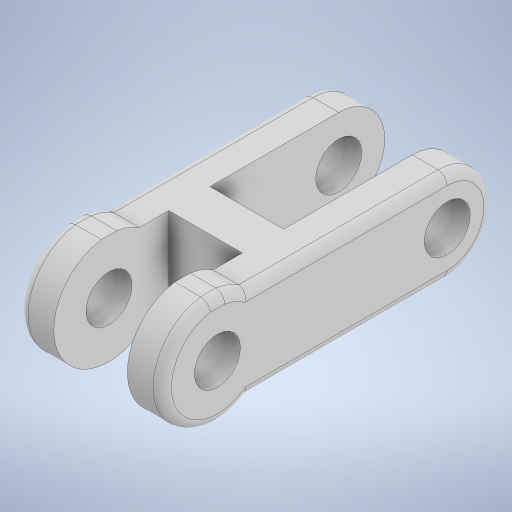
# Autodesk Inventor part: part2
Saved by Autodesk Inventor 2024 (Build 280153000, 153)
## iProperties
Created: 2023-08-22
Part Number: part2
Material: Generic
Document SubType Name: Modeling
Designer: admins
Density: 1 g/cm^3
Appearance: Default
Author: admins
Autodesk Inventor part; units mm, degrees
ref_plane "YZ Plane" through (0, 0, 0) normal (1, 0, 0) x (0, 1, 0)
ref_plane "XZ Plane" through (0, 0, 0) normal (0, 1, 0) x (-1, 0, 0)
ref_plane "XY Plane" through (0, 0, 0) normal (0, 0, 1) x (1, 0, 0)
sketch "Sketch1" plane through (0, 0, 0) normal (0, 1, 0) x (-1, 0, 0)
  line L0 (-138.4477, 131.5515) -> (17.5523, 131.5515)
  line L1 (17.5523, 131.5515) -> (17.5523, -228.4485)
  line L2 (17.5523, -228.4485) -> (-138.4477, -228.4485)
  line L3 (-138.4477, -228.4485) -> (-138.4477, 131.5515)
  point P0 (0, 0)
  dimension "d5" = 156
  dimension "d6" = 360
  constraints: 8 end point, 2 parallel, 1 horizontal, 1 perpendicular
  measures "d5" distance of L1.end L2.end
  measures "d6" distance of L0.end L1.end
extrude "Extrusion2" add sketch "Sketch1" along normal blind 120
sketch "Sketch4" plane through (0, 120, 0) normal (0, 1, 0) x (1, 0, 0)
  line L0 (138.4477, 228.4485) -> (-17.5523, 228.4485) projected
  line L1 (138.4477, 228.4485) -> (100.4477, 228.4485)
  line L2 (100.4477, 228.4485) -> (20.4477, 228.4485)
  line L3 (20.4477, 228.4485) -> (20.4477, 38.4485)
  line L4 (20.4477, 38.4485) -> (100.4477, 38.4485)
  line L5 (100.4477, 38.4485) -> (100.4477, 228.4485)
  point P0 (0, 0)
  dimension "d9" = 38
  dimension "d10" = 80
  dimension "d11" = 190
  constraints: 10 end point, 2 parallel, 1 horizontal, 1 perpendicular, 1 point on line
  measures "d9" distance of L0.start L1.end
  measures "d10" distance of L4.end L3.end
  measures "d11" distance of L3.end L2.end
extrude "Extrusion3" cut sketch "Sketch4" against normal blind 120
sketch "Sketch5" plane through (0, 120, 0) normal (0, 1, 0) x (1, 0, 0)
  line L0 (-17.5523, -131.5515) -> (138.4477, -131.5515) projected
  line L1 (-17.5523, -131.5515) -> (20.4477, -131.5515)
  line L2 (20.4477, -131.5515) -> (100.4477, -131.5515)
  line L3 (100.4477, -131.5515) -> (100.4477, -6.5515)
  line L4 (100.4477, -6.5515) -> (20.4477, -6.5515)
  line L5 (20.4477, -6.5515) -> (20.4477, -131.5515)
  point P0 (0, 0)
  dimension "d14" = 38
  dimension "d15" = 80
  dimension "d16" = 125
  constraints: 10 end point, 2 parallel, 1 horizontal, 1 perpendicular, 1 point on line
  measures "d14" distance of L0.start L1.end
  measures "d15" distance of L4.end L3.end
  measures "d16" distance of L3.end L2.end
extrude "Extrusion4" cut sketch "Sketch5" against normal blind 120
sketch "Sketch6" plane through (-17.5523, 0, -228.4485) normal (-1, 0, 0) x (0, 0, 1)
  circle A0 centre (300, 60.5835) radius 60
  line L0 (360, 0) -> (360, 120) projected
  circle A1 centre (300, 60.5835) radius 25
  circle A2 centre (50, 60.5835) radius 25
  circle A3 centre (50, 60.5835) radius 50
  line L1 (50, 110.5835) -> (266.8338, 110.5835)
  line L2 (50, 10.5835) -> (266.8338, 10.5835)
  line L3 (0, 0) -> (0, 120) projected
  line L4 (0, 120) -> (360, 120)
  line L5 (360, 120) -> (360, 0)
  line L6 (360, 0) -> (0, 0)
  line L7 (0, 0) -> (0, 120)
  point P0 (228.4485, 0)
  point P1 (291.6526, 120)
  point P2 (0, 60.5835)
  point P3 (360, 60.5835)
  point P4 (308.3474, 120)
  dimension "d19" = 120
  dimension "d20" = 50
  dimension "d21" = 50
  dimension "d22" = 250
  dimension "d23" = 100
  constraints: 12 end point, 4 centre point, 4 point on circle, 3 parallel, 2 coincident, 2 horizontal, 1 perpendicular, 1 tangent
  measures "d19" diameter of A0
  measures "d20" diameter of A1
  measures "d21" diameter of A2
  measures "d22" distance of A2.centre A0.centre
  measures "d23" diameter of A3
extrude "Extrusion5" cut sketch "Sketch6" against normal blind 200 contours L1 A3 L3 L4 A0
extrude "Extrusion6" cut sketch "Sketch6" against normal blind 200 contours A0 L0 L6 L3 A3 L2
extrude "Extrusion7" cut sketch "Sketch6" against normal blind 200 contours A0 L4 L0
extrude "Extrusion8" cut sketch "Sketch6" against normal blind 200 contours A2
extrude "Extrusion9" cut sketch "Sketch6" against normal blind 200 contours A1
fillet "Fillet1" radius 10 12 edges at (-17.5523, 60.5835, -228.4485) (-17.5523, 10.5835, -70.0316) (-17.5523, 110.5835, -70.0316) (-17.5523, 116.6815, 50.2675) (-17.5523, 120, 71.5515) (-17.5523, 39.2994, 127.6496) (138.4477, 60.5835, -228.4485) (138.4477, 10.5835, -70.0316) (138.4477, 110.5835, -70.0316) (138.4477, 120, 71.5515) (138.4477, 116.6815, 50.2675) (138.4477, 39.2994, 127.6496)
body "Solid2"
